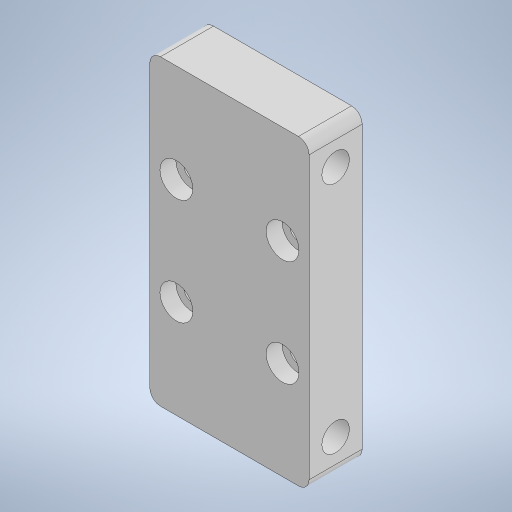
# Autodesk Inventor part: Adapter Mount
Saved by Autodesk Inventor 2023.1 (Build 271208000, 208)
## iProperties
Created: 2023-01-24
Part Number: Adapter Mount
Material: Generic
Document SubType Name: Modeling
Designer: nicol
Density: 1 g/cm^3
Appearance: Default
Author: nicol
Autodesk Inventor part; units mm, degrees
ref_plane "YZ Plane" through (0, 0, 0) normal (1, 0, 0) x (0, 1, 0)
ref_plane "XZ Plane" through (0, 0, 0) normal (0, 1, 0) x (-1, 0, 0)
ref_plane "XY Plane" through (0, 0, 0) normal (0, 0, 1) x (1, 0, 0)
sketch "Sketch1" plane through (0, 0, 0) normal (0, 0, 1) x (1, 0, 0)
  line L0 (-15, 28.5) -> (15, 28.5)
  line L1 (15, 28.5) -> (15, -28.5)
  line L2 (15, -28.5) -> (-15, -28.5)
  line L3 (-15, -28.5) -> (-15, 28.5)
  line L4 (-10, 10) -> (10, 10) construction
  line L5 (10, 10) -> (10, -10) construction
  line L6 (10, -10) -> (-10, -10) construction
  line L7 (-10, -10) -> (-10, 10) construction
  point P0 (0, 0)
  point P1 (0, 10)
  point P2 (0, 28.5)
  point P3 (10, 0)
  point P4 (15, 0)
  dimension "d0" = 20
  dimension "d1" = 30
  dimension "d2" = 57
  constraints: 16 end point, 4 coincident, 4 midpoint, 4 parallel, 3 perpendicular, 2 horizontal, 2 horizontal alignment, 2 vertical alignment
  measures "d0" distance of L4.start L4.end
  measures "d1" distance of L0.start L0.end
  measures "d2" distance of L0.end L1.end
extrude "Extrusion1" add sketch "Sketch1" against normal blind 10
hole "Hole1" at (-10, 10, 0) at (10, 10, 0) at (10, -10, 0) at (-10, -10, 0) direction (0, 0, -1) diameter 3.2 end through all counterbore diameter 6.2 counterbore depth 3
sketch "Sketch2" plane through (15, -28.5, 0) normal (1, 0, 0) x (0, 0, -1)
  line L0 (0, 0) -> (0, 57) projected
  line L1 (0, 0) -> (10, 0) projected
  line L2 (10, 57) -> (10, 0) projected
  line L3 (0, 57) -> (10, 57) projected
  point P0 (0, 28.5)
  point P1 (5, 50.5)
  point P2 (5, 6.5)
  point P3 (5, 57)
  dimension "d12" = 6.5
  dimension "d13" = 6.5
  dimension "d14" = 44
  constraints: 2 vertical alignment, 1 midpoint
  measures "d12" distance from line of L3 point (5, 50.5)
  measures "d13" distance from line of L1 point (5, 6.5)
  measures "d14" distance of point (5, 6.5) point (5, 50.5)
hole "Hole2" at (15, 22, -5) at (15, -22, -5) direction (-1, 0, 0) diameter 5.2 end through all
fillet "Fillet1" radius 2 4 edges at (15, 28.5, -5) (-15, 28.5, -5) (-15, -28.5, -5) (15, -28.5, -5)
equation "\"d13\" = d12"
body "Solid1"
